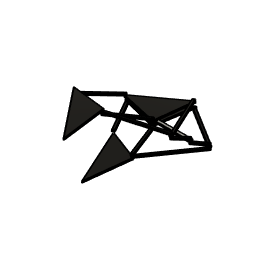
Humanoid leg v8 (Autodesk Fusion 360 design; units mm, degrees)
Autodesk Fusion 360 part; units mm, degrees
sketch "Sketch1" plane through (0, 0, 0) normal (0, 0, 1) x (1, 0, 0) in component "Base"
  line L0 (400, 0) -> (0, 0)
  line L1 (0, 0) -> (0, -70)
  line L2 (0, -70) -> (40, -70)
  line L3 (40, -70) -> (40, -40)
  line L4 (40, -40) -> (400, -40)
  line L5 (400, -40) -> (400, 0)
  circle A0 centre (20, -60) radius 5
  circle A1 centre (390, -20) radius 5
  dimension "d1" = 40
  dimension "d2" = 40
  dimension "d3" = 400
  dimension "d4" = 30
  dimension "d5" = 10
  dimension "d6" = 10
  dimension "d7" = 10
  dimension "d8" = 20
  dimension "d9" = 10
  dimension "d10" = 20
  constraint horizontal L0
  constraint perpendicular L0 L1
  constraint perpendicular L1 L2
  constraint perpendicular L2 L3
  constraint perpendicular L1 L4
  constraint perpendicular L4 L5
  constraint coincident L1.start L0
  constraint coincident L0.end L1.start
  measures "d1" distance of L0.start L4.end
  measures "d2" distance of L1.end L2.end
  measures "d3" distance of L0.start L0.end
  measures "d4" distance of L2.end L3.end
  measures "d5" diameter of A0
  measures "d6" diameter of A1
  measures "d7" distance of L2 A0.centre
  measures "d8" distance of L1 A0.centre
  measures "d9" distance of L5 A1.centre
  measures "d10" distance of L4 A1.centre
extrude "Extrude1" add sketch "Sketch1" along normal blind 20 makes body 1 in component "Base"
sketch "Sketch1 (2)" plane through (0, 0, 0) normal (0, 0, 1) x (1, 0, 0) in component "basecon1"
  circle A0 centre (0, 0) radius 5
  dimension "d13" = 10
  constraint coincident A0.centre origin
  measures "d13" diameter of A0
extrude "Extrude1'" add sketch "Sketch1 (2)" along normal blind 60 separate body makes body 2 in component "basecon1"
fillet "Fillet1" radius 5 6 faces at (400, -26.6667, 6.6667) (266.6667, 0, 6.6667) (0, -23.3333, 6.6667) (13.3333, -70, 6.6667) (160, -40, 6.6667) (40, -60, 6.6667) on bodies 1 in component "Base"
sketch "Sketch1 (3)" plane through (0, 0, 0) normal (0, 0, 1) x (1, 0, 0) in component "l1in"
  line L0 (-100, 30) -> (69, 30)
  line L1 (69, 30) -> (69, 0)
  line L2 (69, 0) -> (-100, 0)
  line L3 (-100, 0) -> (-100, 30)
  circle A0 centre (59, 15) radius 5
  circle A1 centre (-90, 15) radius 5
  dimension "d26" = 30
  dimension "d27" = 169
  dimension "d28" = 10
  dimension "d29" = 10
  dimension "d30" = 10
  dimension "d31" = 10
  dimension "d32" = 15
  dimension "d33" = 15
  constraint horizontal L0
  constraint vertical L1
  constraint horizontal L2
  constraint vertical L3
  measures "d26" distance of L0.end L1.end
  measures "d27" distance of L0.start L0.end
  measures "d28" diameter of A0
  measures "d29" diameter of A1
  measures "d30" distance of L1 A0.centre
  measures "d31" distance of L3 A1.centre
  measures "d32" distance of L2 A1.centre
  measures "d33" distance of L2 A0.centre
extrude "Extrude1''" add sketch "Sketch1 (3)" along normal blind 20 separate body makes body 3 in component "l1in"
fillet "Fillet1'" radius 5 4 faces at (-43.6667, 30, 6.6667) (69, 20, 6.6667) (12.6667, 0, 6.6667) (-100, 10, 6.6667) on bodies 3 in component "l1in"
sketch "Sketch1 (4)" plane through (0, 0, 0) normal (0, 0, 1) x (1, 0, 0) in component "l1 tria"
  line L0 (-328.8444, -265.0736) -> (8.4806, 200.5838)
  line L1 (8.4806, 200.5838) -> (93.2628, -225.0545)
  line L2 (93.2628, -225.0545) -> (-328.8444, -265.0736)
  circle A0 centre (3.1463, 176.1742) radius 5
  circle A1 centre (81.2916, -216.1447) radius 5
  circle A2 centre (-307.7725, -253.031) radius 5
  dimension "d38" = 434
  dimension "d39" = 424
  dimension "d40" = 575
  dimension "d41" = 10
  dimension "d42" = 10
  dimension "d43" = 10
  dimension "d44" = 10
  dimension "d45" = 10
  dimension "d46" = 10
  dimension "d47" = 10
  dimension "d48" = 10
  dimension "d49" = 10
  measures "d38" distance of L0.end L1.end
  measures "d39" distance of L0.start L1.end
  measures "d40" distance of L0.start L0.end
  measures "d41" diameter of A0
  measures "d42" diameter of A1
  measures "d43" diameter of A2
  measures "d44" distance of L0 A0.centre
  measures "d45" distance of L1 A0.centre
  measures "d46" distance of L2 A2.centre
  measures "d47" distance of L0 A2.centre
  measures "d48" distance of L2 A1.centre
  measures "d49" distance of L1 A1.centre
extrude "Extrude1'''" add sketch "Sketch1 (4)" along normal blind 20 separate body makes body 4 in component "l1 tria"
fillet "Fillet1''" radius 5 3 faces at (36.7414, 58.7043, 6.6667) (-216.4027, -109.8545, 6.6667) (-47.4396, -238.3942, 6.6667) on bodies 4 in component "l1 tria"
sketch "Sketch1 (5)" plane through (0, 0, 0) normal (0, 0, 1) x (1, 0, 0) in component "con2"
  circle A0 centre (0, 44) radius 5
  dimension "d54" = 10
  measures "d54" diameter of A0
extrude "Extrude1''''" add sketch "Sketch1 (5)" along normal blind 40 separate body makes body 5 in component "con2"
sketch "Sketch1 (6)" plane through (0, 0, 0) normal (0, 0, 1) x (1, 0, 0) in component "con3"
  circle A0 centre (25, 40) radius 5
  dimension "d57" = 10
  measures "d57" diameter of A0
extrude "Extrude1'''''" add sketch "Sketch1 (6)" along normal blind 60 separate body makes body 6 in component "con3"
sketch "Sketch1 (7)" plane through (0, 0, 0) normal (0, 0, 1) x (1, 0, 0) in component "basecon2"
  circle A0 centre (100, 50) radius 5
  dimension "d64" = 10
  measures "d64" diameter of A0
extrude "Extrude1''''''" add sketch "Sketch1 (7)" along normal blind 100 separate body makes body 7 in component "basecon2"
sketch "Sketch1 (8)" plane through (0, 0, 0) normal (0, 0, 1) x (1, 0, 0) in component "lay2l1"
  line L0 (-150, 100) -> (376, 100)
  line L1 (376, 100) -> (376, 70)
  line L2 (376, 70) -> (-150, 70)
  line L3 (-150, 70) -> (-150, 100)
  circle A0 centre (366, 85) radius 5
  circle A1 centre (-140, 85) radius 5
  dimension "d95" = 30
  dimension "d96" = 526
  dimension "d97" = 10
  dimension "d98" = 10
  dimension "d99" = 10
  dimension "d100" = 10
  constraint horizontal L0
  constraint vertical L1
  constraint horizontal L2
  constraint vertical L3
  measures "d95" distance of L0.end L1.end
  measures "d96" distance of L0.start L0.end
  measures "d97" diameter of A0
  measures "d98" diameter of A1
  measures "d99" distance of L3 A1.centre
  measures "d100" distance of L1 A0.centre
extrude "Extrude1'''''''" add sketch "Sketch1 (8)" along normal blind 20 separate body makes body 8 in component "lay2l1"
fillet "Fillet1'''" radius 5 4 faces at (376, 90, 6.6667) (25.3333, 100, 6.6667) (200.6667, 70, 6.6667) (-150, 80, 6.6667) on bodies 8 in component "lay2l1"
sketch "Sketch1 (9)" plane through (0, 0, 0) normal (0, 0, 1) x (1, 0, 0) in component "lay2l2"
  line L0 (-150, -25) -> (263, -25)
  line L1 (263, -25) -> (263, -55)
  line L2 (263, -55) -> (-150, -55)
  line L3 (-150, -55) -> (-150, -25)
  circle A0 centre (253, -40) radius 5
  circle A1 centre (-140, -40) radius 5
  dimension "d105" = 30
  dimension "d106" = 413
  dimension "d107" = 10
  dimension "d108" = 10
  dimension "d109" = 10
  dimension "d110" = 15
  dimension "d111" = 15
  dimension "d112" = 10
  constraint horizontal L0
  constraint vertical L1
  constraint horizontal L2
  constraint vertical L3
  measures "d105" distance of L0.end L1.end
  measures "d106" distance of L0.start L0.end
  measures "d107" diameter of A0
  measures "d108" diameter of A1
  measures "d109" distance of L3 A1.centre
  measures "d110" distance of L2 A1.centre
  measures "d111" distance of L2 A0.centre
  measures "d112" distance of L1 A0.centre
extrude "Extrude1''''''''" add sketch "Sketch1 (9)" along normal blind 20 separate body makes body 9 in component "lay2l2"
fillet "Fillet1''''" radius 5 4 faces at (-12.3333, -25, 6.6667) (263, -35, 6.6667) (125.3333, -55, 6.6667) (-150, -45, 6.6667) on bodies 9 in component "lay2l2"
sketch "Sketch1 (10)" plane through (0, 0, 0) normal (0, 0, 1) x (1, 0, 0) in component "lay3link"
sketch "Sketch2" plane through (0, 0, 0) normal (0, 0, 1) x (1, 0, 0) in component "lay3link"
  line L0 (-50, 100) -> (575, 100)
  line L1 (575, 100) -> (575, 70)
  line L2 (575, 70) -> (-50, 70)
  line L3 (-50, 70) -> (-50, 100)
  circle A0 centre (-40, 85) radius 5
  circle A1 centre (565, 85) radius 5
  dimension "d142" = 625
  dimension "d143" = 30
  dimension "d144" = 10
  dimension "d145" = 10
  dimension "d146" = 15
  dimension "d147" = 10
  dimension "d148" = 15
  dimension "d149" = 10
  constraint horizontal L0
  constraint vertical L1
  constraint horizontal L2
  constraint vertical L3
  measures "d142" distance of L0.start L0.end
  measures "d143" distance of L0.start L2.end
  measures "d144" diameter of A0
  measures "d145" diameter of A1
  measures "d146" distance of L2 A0.centre
  measures "d147" distance of L3 A0.centre
  measures "d148" distance of L2 A1.centre
  measures "d149" distance of L1 A1.centre
extrude "Extrude1'''''''''" add sketch "Sketch2" along normal blind 20 separate body makes body 10 in component "lay3link"
fillet "Fillet1'''''" radius 5 4 faces at (158.3333, 100, 6.6667) (575, 90, 6.6667) (-50, 80, 6.6667) (366.6667, 70, 6.6667) on bodies 10 in component "lay3link"
sketch "Sketch1 (11)" plane through (0, 0, 0) normal (0, 0, 1) x (1, 0, 0) in component "out"
  line L0 (-250, 250) -> (-419.9412, -89.8823)
  line L1 (-419.9412, -89.8823) -> (257.7859, 137.9576)
  line L2 (257.7859, 137.9576) -> (-250, 250)
  circle A0 centre (-244.5421, 238.5552) radius 5
  circle A1 centre (-400.161, -72.6826) radius 5
  dimension "d162" = 380
  dimension "d163" = 520
  dimension "d164" = 715
  dimension "d166" = 10
  dimension "d167" = 10
  dimension "d168" = 10
  dimension "d169" = 10
  dimension "d172" = 10
  dimension "d173" = 10
  measures "d162" distance of L0.start L0.end
  measures "d163" distance of L0.start L1.end
  measures "d164" distance of L0.end L1.end
  measures "d166" diameter of A0
  measures "d167" diameter of A1
  measures "d168" distance of L0 A1.centre
  measures "d169" distance of L1 A1.centre
  measures "d172" distance of L0 A0.centre
  measures "d173" distance of L2 A0.centre
extrude "Extrude1''''''''''" add sketch "Sketch1 (11)" along normal blind 20 separate body makes body 11 in component "out"
fillet "Fillet1''''''" radius 5 3 faces at (88.5239, 175.3051, 13.3333) (-306.6471, 136.7059, 6.6667) (-194.0321, -13.9357, 6.6667) on bodies 11 in component "out"
ref_plane "WorkPlane1" through (0, 0, 10) normal (0, 0, 1) x (1, 0, 0)
mirror "MirrorComponent1" about plane through (0, 0, 0) normal (0, 0, 1) of bodies 4 makes body 12 in component "l1 tria(Mirror)"
mirror "MirrorComponent1'" about plane through (0, 0, 0) normal (0, 0, 1) of bodies 9 makes body 13 in component "lay2l2(Mirror)"
mirror "MirrorComponent1''" about plane through (0, 0, 0) normal (0, 0, 1) of bodies 11 makes body 14 in component "out(Mirror)"
mirror "MirrorComponent1'''" about plane through (0, 0, 0) normal (0, 0, 1) of bodies 8 makes body 15 in component "lay2l1(Mirror)"
mirror "MirrorComponent1''''" about plane through (0, 0, 0) normal (0, 0, 1) of bodies 3 makes body 16 in component "l1in(Mirror)"
mirror "MirrorComponent1'''''" about plane through (0, 0, 0) normal (0, 0, 1) of bodies 10 makes body 17 in component "lay3link(Mirror)"
component "Base" placed x (1, 0, 0) y (0, 1, 0) z (0, 0, 1) at (0, 0, 0)
component "basecon1" placed x (1, 0, 0) y (0, 1, 0) z (0, 0, 1) at (390, -20, -20)
component "l1in" placed x (0.908168, -0.418606, 0) y (0.418606, 0.908168, 0) z (0, 0, 1) at (330.139, -8.9248, 20)
component "l1 tria" placed x (0.934493, 0.355981, 0) y (-0.355981, 0.934493, 0) z (0, 0, 1) at (-132.9098, 113.0475, 20)
component "con2" placed x (0.934493, 0.355981, 0) y (-0.355981, 0.934493, 0) z (0, 0, 1) at (-177.0211, 237.6834, 20)
component "con3" placed x (0.418606, 0.908168, 0) y (-0.908168, 0.418606, 0) z (0, 0, 1) at (280.5445, 2.9239, 20)
component "basecon2" placed x (1, 0, 0) y (0, 1, 0) z (0, 0, 1) at (-80, -110, -40)
component "con2" placed x (0.934493, 0.355981, 0) y (-0.355981, 0.934493, 0) z (0, 0, 1) at (-314.7838, -274.0871, 20)
component "lay2l1" placed x (0.884125, -0.467251, 0) y (0.467251, 0.884125, 0) z (0, 0, 1) at (-108.6231, 138.2354, 40)
component "lay2l2" placed x (-0.389914, -0.920851, 0) y (0.920851, -0.389914, 0) z (0, 0, 1) at (2.2461, -204.5157, 40)
component "lay2l2" placed x (-0.234802, -0.972043, 0) y (0.972043, -0.234802, 0) z (0, 0, 1) at (-324.4375, -378.4475, 40)
component "con3" placed x (0.920851, -0.389914, 0) y (0.389914, 0.920851, 0) z (0, 0, 1) at (-171.8541, -448.9807, 40)
component "con3" placed x (0.972043, -0.234802, 0) y (0.234802, 0.972043, 0) z (0, 0, 1) at (-456.4174, -647.9941, 40)
component "lay3link" placed x (0.641189, 0.767383, 0) y (-0.767383, 0.641189, 0) z (0, 0, 1) at (-42.3611, -445.7003, 60)
component "out" placed x (0.868357, -0.49594, 0) y (0.49594, 0.868357, 0) z (0, 0, 1) at (-39.1955, -750.3237, 80)
component "l1in(Mirror)" placed x (-0.856437, 0.516251, 0) y (-0.516251, -0.856437, 0) z (0, 0, 1) at (448.2736, -37.6123, 0)
component "l1 tria(Mirror)" placed x (0.787596, -0.616192, 0) y (0.616192, 0.787596, 0) z (0, 0, 1) at (89.1617, 160.3259, 0)
component "lay2l1(Mirror)" placed x (0.627297, -0.77878, 0) y (0.77878, 0.627297, 0) z (0, 0, 1) at (221.8221, 134.7918, -20)
component "lay2l2(Mirror)" placed x (0.021447, -0.99977, 0) y (0.99977, 0.021447, 0) z (0, 0, 1) at (62.9934, -199.1099, -20)
component "lay2l2(Mirror)" placed x (0.164723, -0.98634, 0) y (0.98634, 0.164723, 0) z (0, 0, 1) at (-246.6395, 19.188, -20)
component "lay3link(Mirror)" placed x (0.808563, 0.58841, 0) y (-0.58841, 0.808563, 0) z (0, 0, 1) at (110.7862, -498.101, -40)
component "out(Mirror)" placed x (-0.204451, -0.978877, 0) y (0.978877, -0.204451, 0) z (0, 0, 1) at (-255.0843, -643.5132, -60)
component "con3" placed x (-0.516251, -0.856437, 0) y (0.856437, -0.516251, 0) z (0, 0, 1) at (496.2579, -54.8604, -60)
component "con2" placed x (0.787596, -0.616192, 0) y (0.616192, 0.787596, 0) z (0, 0, 1) at (-336.2668, 116.0324, -40)
component "con2" placed x (0.787596, -0.616192, 0) y (0.616192, 0.787596, 0) z (0, 0, 1) at (173.0843, 262.487, -40)
component "con3" placed x (0.99977, 0.021447, 0) y (-0.021447, 0.99977, 0) z (0, 0, 1) at (4.2925, -493.4366, -80)
component "con3" placed x (0.98634, 0.164723, 0) y (-0.164723, 0.98634, 0) z (0, 0, 1) at (-262.4877, -280.5166, -80)
